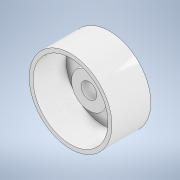
# Autodesk Inventor part: RewingingSpoolBushing
Saved by Autodesk Inventor 2020.2 (Build 242310000, 310)
## iProperties
Created: 2020-03-12
Part Number: RewingingSpoolBushing
Material: Generic
Document SubType Name: Modeling
Designer: elmar
Density: 1 g/cm^3
Appearance: White
Author: elmar
Autodesk Inventor part; units mm, degrees
ref_plane "YZ Plane" through (0, 0, 0) normal (1, 0, 0) x (0, 1, 0)
ref_plane "XY Plane" through (0, 0, 0) normal (0, 0, 1) x (1, 0, 0)
sketch "Sketch1" plane through (0, 0, 0) normal (0, 0, 1) x (1, 0, 0)
  circle A0 centre (0, 0) radius 8.5
  dimension "d0" = 17
  constraints: 1 centre point, 1 coincident
  measures "d0" diameter of A0
extrude "Extrusion1" add sketch "Sketch1" along normal blind 8
sketch "Sketch2" plane through (0, 0, 8) normal (0, 0, 1) x (1, 0, 0)
  circle A0 centre (0, 0) radius 7.7
  circle A1 centre (0, 0) radius 8.5 projected
  dimension "d3" = 0.8
  constraints: 1 centre point, 1 coincident
  measures "d3" radial gap between concentric circles of A1 A0
extrude "Extrusion2" cut sketch "Sketch2" against normal blind 6.8 contours A0
sketch "Sketch3" plane through (0, 0, 0) normal (0, 0, -1) x (-1, 0, 0)
  point P0 (0, 0)
hole "Hole1" at (0, 0, 0) direction (0, 0, 1) diameter 3.2 end through all clearance for "Flat Head Machine Screw" size "M3" standard "Ansi Metric M Profile"
sketch "Sketch4" plane through (0, 0, 1.2) normal (0, 0, 1) x (1, 0, 0)
  circle A0 centre (0, 0) radius 1.6 projected
  circle A1 centre (0, 0) radius 7.7 projected
  line L0 (-11.9, 0) -> (11.9, 0) projected
  line L1 (0, -11.9) -> (0, 11.9) projected
  circle A2 centre (0, 0) radius 3.6
  circle A3 centre (0, 0) radius 4.9
  line L2 (0, 0) -> (2.45, 4.2435)
  line L3 (0, 0) -> (4.2435, 2.45)
  point P0 (0, 7.7)
  point P1 (0, 1.6)
  point P2 (1.6, 0)
  point P3 (7.7, 0)
  point P4 (3.6, 0)
  point P5 (3.1177, 1.8)
  point P6 (4.9, 0)
  point P7 (0, 4.9)
  point P8 (1.8, 3.1177)
  point P9 (0, 3.6)
  dimension "d15" = 30
  dimension "d16" = 30
  dimension "d17" = 9.8
  dimension "d18" = 7.2
  constraints: 4 end point, 2 centre point, 2 coincident, 2 point on circle
  measures "d15" angle of L1 L2
  measures "d16" angle of L0 L3
  measures "d17" diameter of A3
  measures "d18" diameter of A2
extrude "Extrusion3" add sketch "Sketch4" along normal blind 2 contours A0 L3 A2 L0 | A0 L2 A2 L3 | A0 L1 A2 L2 | A2 L2 A3 L3 | A3 L1 A1 L0 picked at (4.6569, 4.8582)
extrude "Extrusion4" add sketch "Sketch4" along normal blind 3 contours L0 A2 L1 A0 | A0 L3 A2 L0 | A0 L2 A2 L3 | L1 A2 L0 A0 | A0 L1 A2 L2 | L0 A2 L1 A0
sketch "Sketch5" plane through (1.8, 3.1177, 1.2) normal (-0.8660254, 0.5, 0) x (0, 0, 1)
  line L0 (0, 0) -> (0, 1.3) projected
  line L1 (0, 0) -> (2, 0) projected
  line L2 (2, 1.3) -> (2, 0) projected
  line L3 (0, 1.3) -> (2, 1.3) projected
  circle A0 centre (0.65, 0.65) radius 0.65
  line L4 (0, 1.3) -> (2, 1.3) projected
  line L5 (0, 0) -> (2, 0) projected
  line L6 (-2.8, -3.6) -> (8.4, -3.6) projected
  point P0 (-1.2, -3.6)
  constraints: 3 tangent, 1 centre point
revolve "Revolution1" cut sketch "Sketch5" angle 10 about axis through (0, 0, -10) along (0, 0, -1) contours A0
ref_plane "Work Plane1" through (0, 0, 0) normal (-0.7071068, 0.7071068, 0) x (0, 0, 1)
mirror "Mirror1" about plane through (0, 0, 0) normal (-0.7071068, 0.7071068, 0) of "Revolution1"
body "Solid1"
